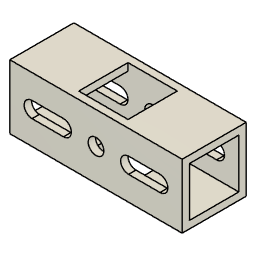
potention_mid_adapter (Autodesk Fusion 360 design; units mm, degrees)
Autodesk Fusion 360 part; units mm, degrees
note: some values were not read from the file. Set by a fixed rule: which sketch regions a step uses.
sketch "スケッチ1" plane through (0, 0, 0) normal (0, 1, 0) x (1, 0, 0)
  line L0 (0, 8) -> (0, -10)
  line L1 (-10, 0) -> (10, 0)
  line L2 (-6.5, 6.5) -> (6.5, 6.5)
  line L3 (6.5, 6.5) -> (6.5, -6.5)
  line L4 (6.5, -6.5) -> (-6.5, -6.5)
  line L5 (-6.5, -6.5) -> (-6.5, 6.5)
  line L6 (-5, 5) -> (5, 5)
  line L7 (5, 5) -> (5, -5)
  line L8 (5, -5) -> (-5, -5)
  line L9 (-5, -5) -> (-5, 5)
  dimension "d1" = 13
  dimension "d2" = 13
  constraint vertical L0
  constraint perpendicular L0 L1
  constraint horizontal L2
  constraint vertical L3
  constraint horizontal L4
  constraint vertical L5
  constraint symmetric L0 L3 L5
  constraint symmetric L1 L2 L4
  constraint horizontal L6
  constraint vertical L7
  constraint horizontal L8
  constraint vertical L9
  measures "d1" distance of L2.start L2.end
  measures "d2" distance of L2.start L4.end
extrude "押し出し1" add sketch "スケッチ1" along normal blind 13 contours L0 L1 L2 L3 L6 L7 | L0 L1 L2 L5 L6 L9 | L0 L1 L4 L5 L8 L9 | L0 L1 L3 L4 L7 L8
sketch "スケッチ2" plane through (0, 0, 6.5) normal (0, 0, 1) x (1, 0, 0)
  line L0 (-6.5, 0) -> (6.5, 0)
  line L1 (6.5, 0) -> (6.5, 13)
  line L2 (6.5, 13) -> (-6.5, 13)
  line L3 (-6.5, 13) -> (-6.5, 0)
  point P0 (0, 6.5)
  dimension "d5" = 6.5
  dimension "d6" = 6.5
  measures "d5" distance of L2 P0
  measures "d6" distance of L3 P0
hole "穴1" at (0, 6.5, 6.5) direction (0, 0, -1) diameter 3.2 depth 20 tip angle 118
sketch "スケッチ3" plane through (6.5, 0, 0) normal (1, 0, 0) x (0, 0, -1)
  line L0 (-6.5, 0) -> (6.5, 0)
  line L1 (6.5, 0) -> (6.5, 13)
  line L2 (6.5, 13) -> (-6.5, 13)
  line L3 (-6.5, 13) -> (-6.5, 0)
  line L4 (-9, 6.5) -> (10, 6.5)
  line L5 (0, 14) -> (0, -2)
  line L6 (-5, 11.5) -> (5, 11.5)
  line L7 (5, 11.5) -> (5, 1.5)
  line L8 (5, 1.5) -> (-5, 1.5)
  line L9 (-5, 1.5) -> (-5, 11.5)
  dimension "d10" = 10
  dimension "d11" = 10
  constraint horizontal L4
  constraint perpendicular L2 L5
  constraint symmetric L0 L2 L4
  constraint symmetric L1 L3 L5
  constraint horizontal L6
  constraint vertical L7
  constraint horizontal L8
  constraint vertical L9
  constraint symmetric L4 L6 L8
  constraint symmetric L5 L7 L9
  measures "d10" distance of L6.start L6.end
  measures "d11" distance of L6.start L8.end
extrude "押し出し2" cut sketch "スケッチ3" against normal blind 17 contours L4 L5 L8 L9 | L4 L5 L7 L8 | L4 L5 L6 L9 | L4 L5 L6 L7
extrude "押し出し3" add 1 faces at (6.5, 4.8333, -6) along direction (1, 0, 0) blind 13
extrude "押し出し4" add 1 faces at (-6.5, 4.8333, 6) along direction (-1, 0, 0) blind 13
sketch "スケッチ4" plane through (0, 13, 0) normal (0, 1, 0) x (-1, 0, 0)
  line L0 (-5, 5) -> (5, 5)
  line L1 (5, 5) -> (5, -5)
  line L2 (5, -5) -> (-5, -5)
  line L3 (-5, -5) -> (-5, 5)
  line L4 (19.5, 6.5) -> (-19.5, 6.5)
  line L5 (-19.5, 6.5) -> (-19.5, -6.5)
  line L6 (-19.5, -6.5) -> (19.5, -6.5)
  line L7 (19.5, -6.5) -> (19.5, 6.5)
sketch "スケッチ5" plane through (0, 0, -6.5) normal (0, 0, -1) x (-1, 0, 0)
  circle A0 centre (0, 6.5) radius 1.6
  line L0 (-19.5, 0) -> (19.5, 0)
  line L1 (19.5, 0) -> (19.5, 13)
  line L2 (19.5, 13) -> (-19.5, 13)
  line L3 (-19.5, 13) -> (-19.5, 0)
  line L4 (-19.5, 13) -> (19.5, 13)
  point P0 (-13, 6.5)
  point P1 (13, 6.5)
  dimension "d18" = 6.5
  dimension "d19" = 6.5
  dimension "d20" = 6.5
  dimension "d21" = 6.5
  measures "d18" distance of L1 P1
  measures "d19" distance of L2 P1
  measures "d20" distance of L3 P0
  measures "d21" distance of P0 L4
hole "穴2" at (13, 6.5, -6.5) at (-13, 6.5, -6.5) direction (0, 0, 1) diameter 3.2 depth 100 tip angle 118
extrude "押し出し5" cut 1 faces at (19.5, 4.8333, -6) along direction (-1, 0, 0) blind 2
extrude "押し出し6" cut 1 faces at (-19.5, 4.8333, 6) along direction (1, 0, 0) blind 2
sketch "スケッチ6" plane through (0, 0, 6.5) normal (0, 0, 1) x (1, 0, 0)
  line L0 (-17.5, 13) -> (-17.5, 0)
  line L1 (-17.5, 0) -> (17.5, 0)
  line L2 (17.5, 0) -> (17.5, 13)
  line L3 (17.5, 13) -> (-17.5, 13)
  circle A0 centre (0, 6.5) radius 1.6
  circle A1 centre (-13, 6.5) radius 1.6
  circle A2 centre (13, 6.5) radius 1.6
  line L4 (-13, 6.5) -> (-9.8, 6.5)
  circle A3 centre (-9.8, 6.5) radius 1.6
  line L5 (13, 6.5) -> (9.8, 6.5)
  circle A4 centre (9.8, 6.5) radius 1.6
  line L6 (-9.8, 6.5) -> (-6.6, 6.5)
  line L7 (9.8, 6.5) -> (6.6, 6.5)
  circle A5 centre (-6.6, 6.5) radius 1.6
  circle A6 centre (6.6, 6.5) radius 1.6
  line L8 (-13, 6.5) -> (-13, 8.1)
  line L9 (-13, 6.5) -> (-13, 4.9)
  line L10 (-13, 8.1) -> (-6.6, 8.1)
  line L11 (-13, 4.9) -> (-6.6, 4.9)
  line L12 (13, 6.5) -> (13, 8.1)
  line L13 (13, 6.5) -> (13, 4.9)
  line L14 (13, 8.1) -> (6.6, 8.1)
  line L15 (13, 4.9) -> (6.6, 4.9)
  dimension "d29" = 3.2
  dimension "d30" = 3.2
  dimension "d31" = 3.2
  dimension "d32" = 3.2
  constraint coincident A1.centre L4.start
  constraint horizontal L4
  constraint coincident L4.end A3.centre
  constraint tangent A1 A3
  constraint coincident A2.centre L5.start
  constraint horizontal L5
  constraint coincident L5.end A4.centre
  constraint tangent A2 A4
  constraint parallel L4 L6
  constraint parallel L3 L7
  constraint coincident L6.end A5.centre
  constraint tangent A3 A5
  constraint coincident L7.end A6.centre
  constraint tangent A4 A6
  constraint coincident A1 L8.end
  constraint perpendicular L4 L8
  constraint coincident A1 L9.end
  constraint perpendicular L4 L9
  constraint coincident A5 L10.end
  constraint tangent A5 L10
  constraint coincident A5 L11.end
  constraint tangent A5 L11
  constraint coincident A2 L12.end
  constraint perpendicular L5 L12
  constraint coincident A2 L13.end
  constraint perpendicular L5 L13
  constraint coincident A6 L14.end
  constraint tangent A6 L14
  constraint coincident A6 L15.end
  constraint tangent A6 L15
  measures "d29" distance of A1.centre L4.end
  measures "d30" distance of A2.centre L5.end
  measures "d31" distance of L4.end L6.end
  measures "d32" distance of L5.end L7.end
extrude "押し出し7" cut sketch "スケッチ6" against normal blind 13 contours A1 A3 L11 | L4 A3 L6 | A1 A3 L10 | L4 A3 L6 | A3 A5 L10 | A3 A5 L11 | A5 | A2 A4 L14 | A2 A4 L15 | L5 A4 L7 | L5 A4 L7 | A4 A6 L14 | A4 A6 L15 | A6
